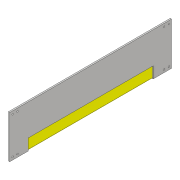
# Autodesk Inventor part: elevatotr
Saved by Autodesk Inventor 2020 (Build 240168000, 168)
## iProperties
Created: 2019-12-24
Part Number: elevatotr
Material: Generic
Document SubType Name: Sheet Metal
Designer: alifhabib
Density: 1 g/cm^3
Sheet Metal Rule: Default_mm
Appearance: Default
Author: alifhabib
Autodesk Inventor part; units mm, degrees
ref_plane "YZ Plane" through (0, 0, 0) normal (1, 0, 0) x (0, 1, 0)
ref_plane "XZ Plane" through (0, 0, 0) normal (0, 1, 0) x (-1, 0, 0)
ref_plane "XY Plane" through (0, 0, 0) normal (0, 0, 1) x (1, 0, 0)
sketch "Sketch1" plane through (0, 0, 0) normal (1, 0, 0) x (0, 1, 0)
  line L0 (75, 285) -> (-75, 285)
  line L1 (-75, 285) -> (-75, -285)
  line L2 (-75, -285) -> (75, -285)
  line L3 (75, -285) -> (75, 285)
  line L4 (75, 285) -> (-75, -285) construction
  line L5 (-75, 285) -> (75, -285) construction
  point P0 (0, 0)
  dimension "d0" = 150
  dimension "d1" = 570
  measures "d0" distance of L2.end L1.end
  measures "d1" distance of L1.end L0.end
extrude "Plate1" add sketch "Sketch1" along normal blind 5
sketch "Sketch2" plane through (5, 0, 0) normal (1, 0, 0) x (0, 0, -1)
  line L0 (-285, 75) -> (-285, -75) projected
  line L1 (-285, -75) -> (-285, -35)
  line L2 (-285, -75) -> (285, -75) projected
  line L3 (0, -75) -> (-220, -75)
  line L4 (0, -75) -> (220, -75)
  line L5 (220, -75) -> (220, -35)
  line L6 (220, -35) -> (0, -35)
  line L7 (0, -35) -> (0, -75)
  line L8 (0, -75) -> (-220, -75)
  line L9 (-220, -75) -> (-220, -35)
  line L10 (-220, -35) -> (0, -35)
  line L11 (0, -35) -> (0, -75)
  point P0 (0, 0)
  dimension "d3" = 40
  dimension "d4" = 220
  dimension "d5" = 220
  dimension "d6" = 40
  dimension "d7" = 220
  dimension "d8" = 40
  constraints: 20 end point, 4 parallel, 2 horizontal, 2 perpendicular, 2 point on line, 1 midpoint
  measures "d3" distance of L0.end L1.end
  measures "d4" distance of L3.start L3.end
  measures "d5" distance of L6.end L5.end
  measures "d6" distance of L5.end L4.end
  measures "d7" distance of L9.end L10.end
  measures "d8" distance of L8.end L9.end
extrude "Cut1" cut sketch "Sketch2" against normal blind 5
sketch "Sketch3" plane through (5, -35, -220) normal (0, -1, 0) x (1, 0, 0)
  line L0 (0, 440) -> (0, 0) projected
  line L1 (0, 440) -> (-5, 440) projected
  line L2 (-5, 0) -> (-5, 440) projected
  line L3 (0, 0) -> (-5, 0) projected
  line L4 (-5, 0) -> (-5, 440) projected
  line L5 (-5, 440) -> (-2, 440)
  line L6 (-2, 440) -> (-2, 0)
  line L7 (-2, 0) -> (-5, 0)
  line L8 (-5, 0) -> (-5, 440)
  point P0 (-5, 220)
  dimension "d11" = 3
  dimension "d12" = 440
  constraints: 8 end point, 2 parallel, 1 horizontal, 1 perpendicular
  measures "d11" distance of L6.end L7.end
  measures "d12" distance of L5.end L6.end
extrude "Extrusion1" add sketch "Sketch3" along normal blind 40 contours L6 L3 L2 L1
fillet "Fillet1" radius 3 1 edges at (3, -75, 0)
sketch "Sketch4" plane through (5, 0, 0) normal (1, 0, 0) x (0, 0, -1)
  line L0 (-285, -75) -> (-285, 75) projected
  line L1 (-220, -75) -> (-285, -75) projected
  circle A0 centre (-275, -65) radius 2.5
  circle A1 centre (-258, -65) radius 2.5
  line L2 (-285, 0) -> (-275, 0)
  circle A2 centre (-275, 65) radius 2.5
  circle A3 centre (-258, 65) radius 2.5
  point P0 (0, 0)
  dimension "d16" = 10
  dimension "d17" = 10
  dimension "d18" = 5
  dimension "d19" = 17
  dimension "d20" = 5
  constraints: 4 centre point, 4 coincident, 4 symmetric about line, 2 end point, 1 horizontal, 1 midpoint, 2 other
  measures "d16" distance from line of L0 point (-275, -65)
  measures "d17" distance from line of L1 point (-275, -65)
  measures "d18" diameter of A0
  measures "d19" distance of A0.centre point (-258, -65)
  measures "d20" diameter of A1
extrude "Extrusion2" cut sketch "Sketch4" against normal mid plane 40
mirror "Mirror1" about plane through (0, 0, 0) normal (0, 0, 1) of "Extrusion2"
equation "\"d9\" = Thickness"
equation "\"d2\" = Thickness"
equation "\"BendRadius\" = Thickness"
equation "\"BendReliefWidth\" = Thickness"
equation "\"BendReliefDepth\" = 0.5 * Thickness"
equation "\"TransitionRadius\" = BendRadius"
equation "\"JacobiRadiusSize\" = BendRadius"
equation "\"GapSize\" = Thickness"
equation "\"Thickness\" = 5"
body "Solid1"
